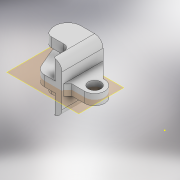
# Autodesk Inventor part: hIP
Saved by Autodesk Inventor 2022 (Build 260153000, 153)
## iProperties
Created: 2022-02-25
Part Number: hIP
Material: Generic
Document SubType Name: Modeling
Designer: joshw
Density: 1 g/cm^3
Appearance: Default
Author: joshw
Autodesk Inventor part; units mm, degrees
ref_plane "YZ Plane" through (0, 0, 0) normal (1, 0, 0) x (0, 1, 0)
ref_plane "XZ Plane" through (0, 0, 0) normal (0, 1, 0) x (-1, 0, 0)
ref_plane "XY Plane" through (0, 0, 0) normal (0, 0, 1) x (1, 0, 0)
sketch "Sketch2" plane through (0, 0, 0) normal (0, 1, 0) x (-1, 0, 0)
  circle A0 centre (25.2851, 7.8895) radius 2.95
  circle A1 centre (25.2851, 7.8895) radius 4.75
  line L0 (25.2851, 3.1395) -> (33.2851, 3.1395)
  line L1 (25.2851, 12.6395) -> (33.2851, 12.6395)
  line L2 (33.2851, 3.1395) -> (33.2851, -4.0935)
  line L3 (33.2851, -4.0935) -> (43.6851, -4.0935)
  arc A2 (43.6851, -4.0935) -> (49.4162, 4.6499) centre (43.6851, 2.1565) ccw
  line L4 (49.4162, 4.6499) -> (44.7437, 15.3895)
  line L5 (44.7437, 15.3895) -> (33.2851, 15.3895)
  line L6 (33.2851, 15.3895) -> (33.2851, 12.6395)
  point P0 (0, 0)
  dimension "d0" = 5.9
  dimension "d1" = 9.5
  dimension "d2" = 8
  dimension "d4" = 10.4
  dimension "d21" = 11.983
  dimension "d22" = 6.25
  constraints: 14 end point, 4 horizontal, 4 point on circle, 4 tangent, 3 centre point, 2 parallel, 2 perpendicular, 1 coincident, 1 point on line, 1 vertical
  measures "d0" diameter of A0
  measures "d1" diameter of A1
  measures "d2" horizontal distance of L0.end A0.centre
  measures "d4" distance of L2.end L3.end
  measures "d21" distance from line of L3 A0.centre
  measures "d22" radius of A2
extrude "Extrusion1" add sketch "Sketch2" along normal mid plane 5
sketch "Sketch4" plane through (0, 2.5, 0) normal (0, 1, 0) x (1, 0, 0)
  line L0 (-33.2851, -3.1395) -> (-33.2851, 4.0935) projected
  line L1 (-44.7437, -15.3895) -> (-33.2851, -15.3895) projected
  line L2 (-33.2851, 4.0935) -> (-37.2851, 4.0935)
  line L3 (-37.2851, 4.0935) -> (-37.2851, -15.3895)
  line L4 (-37.2851, -15.3895) -> (-33.2851, -15.3895)
  line L5 (-33.2851, -15.3895) -> (-33.2851, 4.0935)
  point P0 (0, 0)
  dimension "d8" = 4
  constraints: 8 end point, 2 parallel, 1 horizontal, 1 perpendicular, 1 point on line
  measures "d8" distance of L4.end L3.end
extrude "Extrusion2" add sketch "Sketch4" along normal blind 9.25
sketch "Sketch5" plane through (0, 11.75, 0) normal (0, 1, 0) x (1, 0, 0)
  line L0 (-37.2851, -15.3895) -> (-37.2851, 4.0935) projected
  line L1 (-37.2851, 4.0935) -> (-43.6851, 4.0935) projected
  arc A0 (-43.6851, 4.0935) -> (-49.4162, -4.6499) centre (-43.6851, -2.1565) ccw projected
  line L2 (-49.4162, -4.6499) -> (-44.7437, -15.3895) projected
  line L3 (-44.7437, -15.3895) -> (-37.2851, -15.3895) projected
  point P0 (0, 0)
extrude "Extrusion3" add sketch "Sketch5" against normal blind 4.5
ref_plane "Work Plane1" through (0, 0, 0) normal (0, 1, 0) x (1, 0, 0)
mirror "Mirror1" about plane through (0, 0, 0) normal (0, 1, 0) of "Extrusion2", "Extrusion3"
sketch "Sketch6" plane through (-44.7437, -7.25, 15.3895) normal (0, 1, 0) x (1, 0, 0)
  point P0 (44.7437, 15.3895)
chamfer "Chamfer1" distance 2 angle 45 1 edges at (-33.2851, 0, 12.6395)
fillet "Fillet2" radius 4 2 edges at (-33.2851, 11.75, 5.648) (-33.2851, -11.75, 5.648)
sketch "Sketch7" plane through (-44.7437, -7.25, 15.3895) normal (0, 1, 0) x (1, 0, 0)
  arc A0 (1.0586, 19.483) -> (-4.6725, 10.7396) centre (1.0586, 13.233) ccw projected
  circle A1 centre (0.0586, 12.733) radius 1.75
  circle A2 centre (0.0586, 12.733) radius 6.75
  line L0 (1.0586, 19.483) -> (7.4586, 19.483) projected
  line L1 (1.0586, 19.483) -> (-38.3116, 19.483) construction
  point P0 (44.7437, 15.3895)
  dimension "d18" = 3.5
  dimension "d24" = 13.5
  dimension "d25" = 1
  dimension "d26" = 0.5
  constraints: 3 tangent, 2 centre point, 2 end point, 1 coincident, 1 point on line
  measures "d18" diameter of A1
  measures "d24" diameter of A2
  measures "d25" horizontal distance of A1.centre A0.centre
  measures "d26" vertical distance of A0.centre A1.centre
extrude "Extrusion4" add sketch "Sketch7" along normal up to surface (14.5 mm away) contours A1
sketch "Sketch8" plane through (0, 11.75, 0) normal (0, 1, 0) x (1, 0, 0)
  line L0 (-54.2603, -7.4065) -> (-37.2851, -7.4065)
  line L1 (-37.2851, -7.4065) -> (-37.2851, -23.5954)
  line L2 (-37.2851, 4.0935) -> (-37.2851, -15.3895) projected
  line L3 (-37.2851, 4.0935) -> (-43.6851, 4.0935) projected
  arc A0 (-43.6851, 4.0935) -> (-49.4162, -4.6499) centre (-43.6851, -2.1565) ccw projected
  line L4 (-49.4162, -4.6499) -> (-44.7437, -15.3895) projected
  line L5 (-44.7437, -15.3895) -> (-37.2851, -15.3895) projected
  point P0 (0, 0)
  point P1 (-48.2169, -7.4065)
  dimension "d28" = 11.5
  constraints: 4 end point, 1 collinear, 1 horizontal, 1 perpendicular
  measures "d28" distance between parallel lines of L3 L0
extrude "Extrusion5" cut sketch "Sketch8" against normal up to surface (4.5 mm away) contours L0 L1 L5 L4
mirror "Mirror2" about plane through (0, 0, 0) normal (0, 1, 0) of "Extrusion5"
fillet "Fillet3" radius 3 2 edges at (-48.2169, 9.5, 7.4065) (-37.2851, 9.5, 7.4065)
fillet "Fillet4" radius 3 2 edges at (-48.2169, -9.5, 7.4065) (-37.2851, -9.5, 7.4065)
fillet "Fillet5" radius 5 1 edges at (-44.7437, 0, 15.3895)
fillet "Fillet6" radius 1 2 edges at (-37.2851, 7.125, 15.3895) (-37.2851, -7.125, 15.3895)
chamfer "Chamfer2" distance 7.23 angle 45 1 edges at (-33.2851, 0, 3.1395)
body "Solid1"
